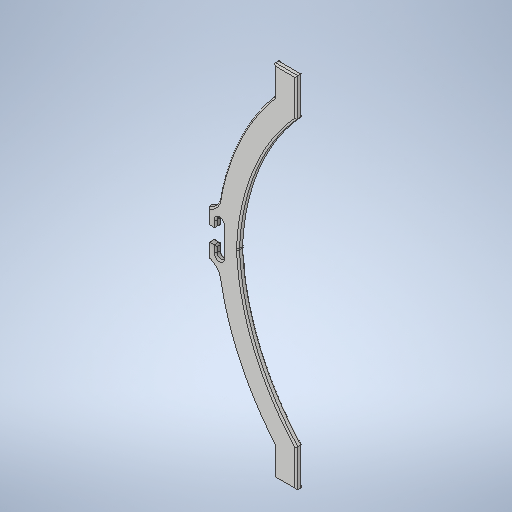
# Autodesk Inventor part: Baseplate_aussen
Saved by Autodesk Inventor 2025 (Build 290162000, 162)
## iProperties
Created: 2020-01-15
Part Number: Baseplate_aussen
Material: Generisch
Document SubType Name: Modeling
Designer: maxse
Density: 1 g/cm^3
Appearance: Vorgabe
Author: maxse
Autodesk Inventor part; units mm, degrees
(part 1 of 2)
ref_plane "YZ Plane" through (0, 0, 0) normal (1, 0, 0) x (0, 1, 0)
ref_plane "XZ Plane" through (0, 0, 0) normal (0, 1, 0) x (-1, 0, 0)
ref_plane "XY Plane" through (0, 0, 0) normal (0, 0, 1) x (1, 0, 0)
sketch "Skizze1" plane through (0, 0, 0) normal (0, 1, 0) x (-1, 0, 0)
  arc A0 (39, 0) -> (0, 95) centre (-110.879, -6.024) ccw
  line L0 (0, 95) -> (0, 120)
  line L1 (0, 120) -> (15, 120)
  line L2 (15, 120) -> (15, 100.6336)
  arc A1 (54, 0) -> (15, 100.6336) centre (-110.879, -6.024) ccw
  line L3 (39, 0) -> (54, 0)
  line L4 (0, 0) -> (39, 0)
  line L5 (59, 0) -> (59, 15)
  line L6 (59, 15) -> (52.765, 15)
  line L7 (59, 0) -> (54, 0)
  dimension "d0" = 25
  dimension "d2" = 15
  dimension "d4" = 54
  dimension "d5" = 0
  dimension "d6" = 120
  dimension "d7" = 150
  dimension "d9" = 5
  dimension "d10" = 15
  dimension "d11" = 15
  constraints: 16 end point, 6 point on circle, 3 perpendicular, 2 centre point, 2 horizontal, 2 vertical, 1 collinear, 1 concentric
  measures "d0" distance of L0.start L0.end
  measures "d2" distance of L0.end L1.end
  measures "d4" distance of L3.end L4.start
  measures "d5" distance from line of L4.start L0
  measures "d6" distance from line of L4.start L1
  measures "d7" radius of A0
  measures "d9" distance of L3.end L5.start
  measures "d10" distance of L3.end L3.start
  measures "d11" distance of L5.start L5.end
extrude "Extrusion1" add sketch "Skizze1" along normal blind 4
mirror "Spiegeln1" about plane through (-54, 0, 0) normal (0, 0, -1) of "Extrusion1"
sketch "Skizze2" plane through (0, 0, 0) normal (0, -1, 0) x (1, 0, 0)
  line L0 (-59, 15) -> (-59, -15) projected
  line L1 (-59, -5) -> (-54, -5)
  line L2 (-54, -5) -> (-54, -9.5)
  line L3 (-59, 5) -> (-54, 5)
  line L4 (-54, 5) -> (-54, 9.5)
  line L5 (-49, -9.5) -> (-49, 9.5)
  arc A0 (-49, 9.5) -> (-54, 9.5) centre (-51.5, 9.5) ccw
  arc A1 (-54, -9.5) -> (-49, -9.5) centre (-51.5, -9.5) ccw
  point P0 (0, 0)
  dimension "d15" = 10
  dimension "d16" = 5
  dimension "d17" = 10
  dimension "d18" = 5
  dimension "d19" = 5
  dimension "d20" = 24
  dimension "d21" = 4.5
  constraints: 10 end point, 4 point on circle, 4 tangent, 2 centre point, 2 horizontal, 2 point on line, 2 vertical, 1 perpendicular
  measures "d15" distance between parallel lines of L5 L0
  measures "d16" distance between parallel lines of L5 L2
  measures "d17" distance between parallel lines of L3 L1
  measures "d18" distance of L3.start L3.end
  measures "d19" distance from line of point (0, 0) L3
  measures "d21" distance from line of L1 A1.centre
extrude "Extrusion2" cut sketch "Skizze2" against normal blind 4
fillet "Rundung1" radius 10 3 edges at (-52.765, 2, -15) (-52.765, 2, 15) (-39, 2, 0)
fillet "Rundung2" radius 1 46 edges at (-7.5, 4, -120) (0, 4, -107.5) (-15, 4, -110.3168) (-7.5, 0, -120) (0, 0, -107.5) (-15, 0, -110.3168) (-54.0935, 4, -17.8718) (-38.4134, 4, -64.2123) (-54.0935, 0, -17.8718) (-38.4134, 0, -64.2123) (-38.9913, 4, 0) (-27.8012, 4, 51.1406) (-27.8012, 4, -51.1406) (-38.9913, 0, 0) (-27.8012, 0, 51.1406) (-27.8012, 0, -51.1406) (-54.0935, 4, 17.8718) (-38.4134, 4, 64.2123) (-54.0935, 0, 17.8718) (-38.4134, 0, 64.2123) (-59, 4, 10) (-59, 0, 10) (-59, 0, -10) (-59, 4, -10) (-59, 2, -5) (-59, 2, 5) (-54, 2, 5) (-54, 2, -5) (-56.5, 4, -5) (-56.5, 4, 5) (-51.5, 4, 12) (-54, 4, 7.25) (-51.5, 4, -12) (-54, 4, -7.25) (-49, 4, 0) (-51.5, 0, -12) (-54, 0, -7.25) (-51.5, 0, 12) (-54, 0, 7.25) (-49, 0, 0) (-15, 4, 110.3168) (-15, 0, 110.3168) (-7.5, 4, 120) (-7.5, 0, 120) (0, 0, 107.5) (0, 4, 107.5)
sketch "Skizze3" plane through (0, 4, 0) normal (0, 1, 0) x (1, 0, 0)
  line L0 (0, 120) -> (0, 95) projected
  arc A0 (0, 95) -> (0, -95.3865) centre (95.1198, -0.1933) ccw
  line L1 (-30.1986, 63.5083) -> (-29.9063, 64.0688)
  line L2 (-29.9063, 64.0688) -> (-28.0095, 63.0792)
  spline S0 degree 2 poles (-28.0095, 63.0792) (-27.7796, 62.9593) (-27.3619, 62.7962) (-27.2096, 62.799) knots 0 0 0 1 2 2 2
  spline S1 degree 2 poles (-27.2096, 62.799) (-27.0483, 62.8017) (-26.7987, 62.9822) (-26.69, 63.1906) knots 0 0 0 1 2 2 2
  spline S2 degree 2 poles (-26.69, 63.1906) (-26.5813, 63.399) (-26.5735, 63.957) (-26.6426, 64.2627) knots 0 0 0 1 2 2 2
  line L3 (-26.6426, 64.2627) -> (-29.1285, 65.5596)
  line L4 (-29.1285, 65.5596) -> (-28.8361, 66.12)
  line L5 (-28.8361, 66.12) -> (-24.2056, 63.7042)
  line L6 (-24.2056, 63.7042) -> (-24.4979, 63.1438)
  line L7 (-24.4979, 63.1438) -> (-26.172, 64.0172)
  spline S3 degree 2 poles (-26.172, 64.0172) (-26.0768, 63.6476) (-26.0928, 63.039) (-26.2352, 62.7659) knots 0 0 0 1 2 2 2
  spline S4 degree 2 poles (-26.2352, 62.7659) (-26.4901, 62.2774) (-27.4253, 62.0615) (-28.0396, 62.382) knots 0 0 0 1 2 2 2
  line L8 (-28.0396, 62.382) -> (-30.1986, 63.5083)
  spline S5 degree 2 poles (-30.2636, 59.1219) (-31.1157, 59.5377) (-31.6445, 60.8101) (-31.3105, 61.4947) knots 0 0 0 1 2 2 2
  spline S6 degree 2 poles (-31.3105, 61.4947) (-30.9676, 62.1975) (-29.6172, 62.535) (-28.7942, 62.1334) knots 0 0 0 1 2 2 2
  spline S7 degree 2 poles (-28.7942, 62.1334) (-27.9494, 61.7212) (-27.4186, 60.4343) (-27.7491, 59.757) knots 0 0 0 1 2 2 2
  spline S8 degree 2 poles (-27.7491, 59.757) (-28.0831, 59.0724) (-29.4152, 58.7079) (-30.2636, 59.1219) knots 0 0 0 1 2 2 2
  spline S9 degree 2 poles (-29.9776, 59.7082) (-29.3221, 59.3884) (-28.4521, 59.5545) (-28.2371, 59.9951) knots 0 0 0 1 2 2 2
  spline S10 degree 2 poles (-28.2371, 59.9951) (-28.0221, 60.4357) (-28.4248, 61.2273) (-29.0803, 61.5471) knots 0 0 0 1 2 2 2
  spline S11 degree 2 poles (-29.0803, 61.5471) (-29.7175, 61.8581) (-30.6075, 61.6972) (-30.8225, 61.2566) knots 0 0 0 1 2 2 2
  spline S12 degree 2 poles (-30.8225, 61.2566) (-31.0357, 60.8196) (-30.6257, 60.0245) (-29.9776, 59.7082) knots 0 0 0 1 2 2 2
  line L9 (-32.4885, 58.7697) -> (-32.222, 59.3429)
  line L10 (-32.222, 59.3429) -> (-27.4858, 57.1415)
  line L11 (-27.4858, 57.1415) -> (-27.7522, 56.5683)
  line L12 (-27.7522, 56.5683) -> (-32.4885, 58.7697)
  line L13 (-34.047, 55.2901) -> (-33.7916, 55.8683)
  line L14 (-33.7916, 55.8683) -> (-33.4432, 55.7144)
  spline S13 degree 2 poles (-33.4432, 55.7144) (-33.4954, 55.897) (-33.5569, 56.1589) (-33.561, 56.3202) knots 0 0 0 1 2 2 2
  spline S14 degree 2 poles (-33.561, 56.3202) (-33.5663, 56.4687) (-33.513, 56.7596) (-33.4361, 56.9338) knots 0 0 0 1 2 2 2
  spline S15 degree 2 poles (-33.4361, 56.9338) (-33.3116, 57.2155) (-32.8686, 57.5868) (-32.5688, 57.6537) knots 0 0 0 1 2 2 2
  spline S16 degree 2 poles (-32.5688, 57.6537) (-32.269, 57.7206) (-31.52, 57.6112) (-31.0864, 57.4196) knots 0 0 0 1 2 2 2
  spline S17 degree 2 poles (-31.0864, 57.4196) (-30.6342, 57.2199) (-30.0776, 56.695) (-29.9194, 56.3814) knots 0 0 0 1 2 2 2
  spline S18 degree 2 poles (-29.9194, 56.3814) (-29.7805, 56.0942) (-29.7589, 55.4512) (-29.8882, 55.1584) knots 0 0 0 1 2 2 2
  spline S19 degree 2 poles (-29.8882, 55.1584) (-30.0012, 54.9026) (-30.2847, 54.5716) (-30.4967, 54.4128) knots 0 0 0 1 2 2 2
  line L15 (-30.4967, 54.4128) -> (-29.0141, 53.7579)
  line L16 (-29.0141, 53.7579) -> (-29.2696, 53.1797)
  line L17 (-29.2696, 53.1797) -> (-34.047, 55.2901)
  line L18 (-32.9577, 55.4999) -> (-30.9748, 54.624)
  spline S20 degree 2 poles (-30.9748, 54.624) (-30.776, 54.7931) (-30.5476, 55.0997) (-30.4608, 55.2961) knots 0 0 0 1 2 2 2
  spline S21 degree 2 poles (-30.4608, 55.2961) (-30.2643, 55.7409) (-30.7088, 56.5397) (-31.3389, 56.818) knots 0 0 0 1 2 2 2
  spline S22 degree 2 poles (-31.3389, 56.818) (-31.9467, 57.0865) (-32.7582, 56.9843) (-32.9465, 56.5581) knots 0 0 0 1 2 2 2
  spline S23 degree 2 poles (-32.9465, 56.5581) (-33.0463, 56.332) (-33.0418, 55.7807) (-32.9577, 55.4999) knots 0 0 0 1 2 2 2
  spline S24 degree 2 poles (-35.1022, 52.9728) (-34.7605, 53.8049) (-33.4517, 54.3363) (-32.5896, 53.9824) knots 0 0 0 1 2 2 2
  spline S25 degree 2 poles (-32.5896, 53.9824) (-31.7425, 53.6346) (-31.1027, 52.3338) (-31.3967, 51.6179) knots 0 0 0 1 2 2 2
  spline S26 degree 2 poles (-31.3967, 51.6179) (-31.529, 51.2955) (-31.9211, 50.874) (-32.1952, 50.7719) knots 0 0 0 1 2 2 2
  spline S27 degree 2 poles (-32.1952, 50.7719) (-32.4708, 50.666) (-33.1258, 50.7028) (-33.5419, 50.8736) knots 0 0 0 1 2 2 2
  line L19 (-33.5419, 50.8736) -> (-33.8605, 51.0044)
  line L20 (-33.8605, 51.0044) -> (-32.874, 53.4071)
  spline S28 degree 2 poles (-32.874, 53.4071) (-33.4775, 53.6548) (-34.3677, 53.3108) (-34.5894, 52.771) knots 0 0 0 1 2 2 2
  spline S29 degree 2 poles (-34.5894, 52.771) (-34.6678, 52.5799) (-34.734, 52.1734) (-34.7281, 51.9958) knots 0 0 0 1 2 2 2
  spline S30 degree 2 poles (-34.7281, 51.9958) (-34.7177, 51.8076) (-34.6758, 51.5363) (-34.6451, 51.4405) knots 0 0 0 1 2 2 2
  line L21 (-34.6451, 51.4405) -> (-34.6589, 51.4067)
  line L22 (-34.6589, 51.4067) -> (-35.2961, 51.6684)
  spline S31 degree 2 poles (-35.2961, 51.6684) (-35.2958, 51.7865) (-35.2896, 52.1431) (-35.274, 52.2769) knots 0 0 0 1 2 2 2
  spline S32 degree 2 poles (-35.274, 52.2769) (-35.2535, 52.4656) (-35.1884, 52.7629) (-35.1022, 52.9728) knots 0 0 0 1 2 2 2
  spline S33 degree 2 poles (-33.1805, 51.391) (-32.9413, 51.3016) (-32.5565, 51.2575) (-32.4018, 51.3035) knots 0 0 0 1 2 2 2
  spline S34 degree 2 poles (-32.4018, 51.3035) (-32.229, 51.3508) (-31.9596, 51.6125) (-31.8626, 51.8486) knots 0 0 0 1 2 2 2
  spline S35 degree 2 poles (-31.8626, 51.8486) (-31.7672, 52.081) (-31.772, 52.464) (-31.8515, 52.6544) knots 0 0 0 1 2 2 2
  spline S36 degree 2 poles (-31.8515, 52.6544) (-31.9363, 52.8425) (-32.2145, 53.1144) (-32.428, 53.2239) knots 0 0 0 1 2 2 2
  line L23 (-32.428, 53.2239) -> (-33.1805, 51.391)
  line L24 (-33.6101, 48.1318) -> (-33.5984, 48.162)
  spline S37 degree 2 poles (-33.5984, 48.162) (-33.5533, 48.2228) (-33.4889, 48.3673) (-33.4495, 48.4694) knots 0 0 0 1 2 2 2
  spline S38 degree 2 poles (-33.4495, 48.4694) (-33.3577, 48.7076) (-33.385, 49.2565) (-33.5075, 49.547) knots 0 0 0 1 2 2 2
  line L25 (-33.5075, 49.547) -> (-35.9915, 50.5044)
  line L26 (-35.9915, 50.5044) -> (-35.7641, 51.0942)
  line L27 (-35.7641, 51.0942) -> (-32.2632, 49.7447)
  line L28 (-32.2632, 49.7447) -> (-32.4905, 49.1549)
  line L29 (-32.4905, 49.1549) -> (-33.0122, 49.3561)
  spline S39 degree 2 poles (-33.0122, 49.3561) (-32.8488, 48.9239) (-32.7995, 48.3534) (-32.8869, 48.1266) knots 0 0 0 1 2 2 2
  spline S40 degree 2 poles (-32.8869, 48.1266) (-32.9219, 48.0359) (-32.9644, 47.948) (-32.9976, 47.8957) knots 0 0 0 1 2 2 2
  line L30 (-32.9976, 47.8957) -> (-33.6101, 48.1318)
  line L31 (-33.6727, 43.3761) -> (-33.662, 43.4067)
  spline S41 degree 2 poles (-33.662, 43.4067) (-33.6034, 43.4764) (-33.4458, 43.7561) (-33.4044, 43.8747) knots 0 0 0 1 2 2 2
  spline S42 degree 2 poles (-33.4044, 43.8747) (-33.2737, 44.2497) (-33.4983, 44.6884) (-33.9421, 44.8432) knots 0 0 0 1 2 2 2
  line L32 (-33.9421, 44.8432) -> (-34.0607, 44.8845)
  line L33 (-34.0607, 44.8845) -> (-34.4049, 43.8975)
  line L34 (-34.4049, 43.8975) -> (-34.8985, 44.0695)
  line L35 (-34.8985, 44.0695) -> (-34.5609, 45.0375)
  line L36 (-34.5609, 45.0375) -> (-37.6102, 46.1008)
  line L37 (-37.6102, 46.1008) -> (-37.4021, 46.6976)
  line L38 (-37.4021, 46.6976) -> (-34.3528, 45.6344)
  line L39 (-34.3528, 45.6344) -> (-34.2127, 46.0361)
  line L40 (-34.2127, 46.0361) -> (-33.7192, 45.864)
  line L41 (-33.7192, 45.864) -> (-33.8593, 45.4623)
  line L42 (-33.8593, 45.4623) -> (-33.7407, 45.4209)
  spline S43 degree 2 poles (-33.7407, 45.4209) (-33.1056, 45.1995) (-32.6546, 44.3514) (-32.8547, 43.7775) knots 0 0 0 1 2 2 2
  spline S44 degree 2 poles (-32.8547, 43.7775) (-32.9121, 43.6129) (-33.0573, 43.3074) (-33.1256, 43.1853) knots 0 0 0 1 2 2 2
  line L43 (-33.1256, 43.1853) -> (-33.6727, 43.3761)
  spline S45 degree 2 poles (-37.3148, 41.0423) (-38.2166, 41.335) (-38.9178, 42.5212) (-38.6826, 43.2457) knots 0 0 0 1 2 2 2
  spline S46 degree 2 poles (-38.6826, 43.2457) (-38.4411, 43.9895) (-37.151, 44.5122) (-36.28, 44.2294) knots 0 0 0 1 2 2 2
  spline S47 degree 2 poles (-36.28, 44.2294) (-35.386, 43.9391) (-34.6808, 42.7389) (-34.9135, 42.0221) knots 0 0 0 1 2 2 2
  spline S48 degree 2 poles (-34.9135, 42.0221) (-35.1488, 41.2975) (-36.4169, 40.7507) (-37.3148, 41.0423) knots 0 0 0 1 2 2 2
  spline S49 degree 2 poles (-37.1134, 41.6627) (-36.4197, 41.4375) (-35.5813, 41.7234) (-35.4299, 42.1897) knots 0 0 0 1 2 2 2
  spline S50 degree 2 poles (-35.4299, 42.1897) (-35.2785, 42.656) (-35.7878, 43.3837) (-36.4815, 43.6089) knots 0 0 0 1 2 2 2
  spline S51 degree 2 poles (-36.4815, 43.6089) (-37.1559, 43.8279) (-38.0148, 43.5444) (-38.1662, 43.0781) knots 0 0 0 1 2 2 2
  spline S52 degree 2 poles (-38.1662, 43.0781) (-38.3163, 42.6156) (-37.7993, 41.8854) (-37.1134, 41.6627) knots 0 0 0 1 2 2 2
  line L44 (-36.9101, 38.2097) -> (-36.9008, 38.2408)
  spline S53 degree 2 poles (-36.9008, 38.2408) (-36.8604, 38.3048) (-36.8072, 38.4538) (-36.7757, 38.5586) knots 0 0 0 1 2 2 2
  spline S54 degree 2 poles (-36.7757, 38.5586) (-36.7023, 38.8031) (-36.7711, 39.3484) (-36.9154, 39.6286) knots 0 0 0 1 2 2 2
  line L45 (-36.9154, 39.6286) -> (-39.4649, 40.3945)
  line L46 (-39.4649, 40.3945) -> (-39.2831, 40.9999)
  line L47 (-39.2831, 40.9999) -> (-35.6897, 39.9204)
  line L48 (-35.6897, 39.9204) -> (-35.8715, 39.315)
  line L49 (-35.8715, 39.315) -> (-36.4071, 39.4759)
  spline S55 degree 2 poles (-36.4071, 39.4759) (-36.2112, 39.0575) (-36.1187, 38.4923) (-36.1886, 38.2595) knots 0 0 0 1 2 2 2
  spline S56 degree 2 poles (-36.1886, 38.2595) (-36.2166, 38.1664) (-36.2524, 38.0756) (-36.2815, 38.0209) knots 0 0 0 1 2 2 2
  line L50 (-36.2815, 38.0209) -> (-36.9101, 38.2097)
  spline S57 degree 2 poles (-41.0374, 35.2117) (-40.9436, 35.5725) (-40.574, 36.1085) (-40.3199, 36.2644) knots 0 0 0 1 2 2 2
  spline S58 degree 2 poles (-40.3199, 36.2644) (-40.0708, 36.4173) (-39.4825, 36.4904) (-39.1805, 36.4118) knots 0 0 0 1 2 2 2
  spline S59 degree 2 poles (-39.1805, 36.4118) (-38.7884, 36.3099) (-38.2387, 35.719) (-38.1466, 35.268) knots 0 0 0 1 2 2 2
  line L51 (-38.1466, 35.268) -> (-38.127, 35.2629)
  spline S60 degree 2 poles (-38.127, 35.2629) (-37.8264, 35.5657) (-37.2425, 35.7823) (-36.8739, 35.6865) knots 0 0 0 1 2 2 2
  spline S61 degree 2 poles (-36.8739, 35.6865) (-36.3288, 35.5447) (-35.8136, 34.5316) (-35.9788, 33.8963) knots 0 0 0 1 2 2 2
  spline S62 degree 2 poles (-35.9788, 33.8963) (-36.1501, 33.2375) (-37.0472, 32.6209) (-37.5884, 32.7616) knots 0 0 0 1 2 2 2
  spline S63 degree 2 poles (-37.5884, 32.7616) (-37.9139, 32.8462) (-38.4502, 33.3918) (-38.5378, 33.7956) knots 0 0 0 1 2 2 2
  line L52 (-38.5378, 33.7956) -> (-38.5574, 33.8007)
  spline S64 degree 2 poles (-38.5574, 33.8007) (-38.8636, 33.4281) (-39.5415, 33.1397) (-39.9886, 33.2559) knots 0 0 0 1 2 2 2
  spline S65 degree 2 poles (-39.9886, 33.2559) (-40.6082, 33.417) (-41.2128, 34.5372) (-41.0374, 35.2117) knots 0 0 0 1 2 2 2
  spline S66 degree 2 poles (-39.878, 33.9389) (-39.5799, 33.8614) (-39.1658, 34.0049) (-38.8988, 34.2913) knots 0 0 0 1 2 2 2
  spline S67 degree 2 poles (-38.8988, 34.2913) (-38.8075, 34.3848) (-38.5665, 34.7157) (-38.4122, 34.9226) knots 0 0 0 1 2 2 2
  spline S68 degree 2 poles (-38.4122, 34.9226) (-38.5194, 35.2351) (-38.9704, 35.6581) (-39.3037, 35.7447) knots 0 0 0 1 2 2 2
  spline S69 degree 2 poles (-39.3037, 35.7447) (-39.7429, 35.8589) (-40.4531, 35.4784) (-40.5571, 35.0784) knots 0 0 0 1 2 2 2
  spline S70 degree 2 poles (-40.5571, 35.0784) (-40.6632, 34.6706) (-40.3015, 34.049) (-39.878, 33.9389) knots 0 0 0 1 2 2 2
  spline S71 degree 2 poles (-37.4311, 33.3989) (-37.1056, 33.3143) (-36.5571, 33.6364) (-36.4562, 34.0246) knots 0 0 0 1 2 2 2
  spline S72 degree 2 poles (-36.4562, 34.0246) (-36.3644, 34.3775) (-36.6353, 34.9295) (-36.9687, 35.0161) knots 0 0 0 1 2 2 2
  spline S73 degree 2 poles (-36.9687, 35.0161) (-37.2079, 35.0783) (-37.6014, 34.9336) (-37.7948, 34.7369) knots 0 0 0 1 2 2 2
  spline S74 degree 2 poles (-37.7948, 34.7369) (-37.8752, 34.6532) (-38.1755, 34.2875) (-38.2742, 34.1331) knots 0 0 0 1 2 2 2
  spline S75 degree 2 poles (-38.2742, 34.1331) (-38.132, 33.7947) (-37.7252, 33.4754) (-37.4311, 33.3989) knots 0 0 0 1 2 2 2
  spline S76 degree 2 poles (-40.6166, 29.5675) (-40.9916, 29.6544) (-41.5695, 30.0503) (-41.7342, 30.3089) knots 0 0 0 1 2 2 2
  spline S77 degree 2 poles (-41.7342, 30.3089) (-41.9089, 30.5782) (-42.0155, 31.1769) (-41.9396, 31.5045) knots 0 0 0 1 2 2 2
  spline S78 degree 2 poles (-41.9396, 31.5045) (-41.8637, 31.8321) (-41.5173, 32.3217) (-41.2487, 32.4757) knots 0 0 0 1 2 2 2
  spline S79 degree 2 poles (-41.2487, 32.4757) (-40.9257, 32.667) (-39.9717, 32.7454) (-39.3244, 32.5954) knots 0 0 0 1 2 2 2
  spline S80 degree 2 poles (-39.3244, 32.5954) (-38.6888, 32.4482) (-37.7269, 31.9508) (-37.411, 31.5906) knots 0 0 0 1 2 2 2
  spline S81 degree 2 poles (-37.411, 31.5906) (-37.1013, 31.2401) (-36.8807, 30.3073) (-37.0079, 29.7586) knots 0 0 0 1 2 2 2
  spline S82 degree 2 poles (-37.0079, 29.7586) (-37.0454, 29.5968) (-37.1428, 29.3199) (-37.203, 29.2215) knots 0 0 0 1 2 2 2
  line L53 (-37.203, 29.2215) -> (-37.8307, 29.367)
  line L54 (-37.8307, 29.367) -> (-37.8243, 29.3946)
  spline S83 degree 2 poles (-37.8243, 29.3946) (-37.7558, 29.4744) (-37.5961, 29.7868) (-37.5522, 29.9762) knots 0 0 0 1 2 2 2
  spline S84 degree 2 poles (-37.5522, 29.9762) (-37.4114, 30.5841) (-38.0595, 31.5204) (-38.8483, 31.7781) knots 0 0 0 1 2 2 2
  spline S85 degree 2 poles (-38.8483, 31.7781) (-38.7404, 31.5077) (-38.6762, 30.977) (-38.7439, 30.6849) knots 0 0 0 1 2 2 2
  spline S86 degree 2 poles (-38.7439, 30.6849) (-38.8098, 30.4007) (-39.023, 30.001) (-39.2507, 29.8083) knots 0 0 0 1 2 2 2
  spline S87 degree 2 poles (-39.2507, 29.8083) (-39.5142, 29.5865) (-40.1982, 29.4705) (-40.6166, 29.5675) knots 0 0 0 1 2 2 2
  spline S88 degree 2 poles (-40.4906, 30.237) (-40.1906, 30.1675) (-39.7474, 30.2312) (-39.5651, 30.372) knots 0 0 0 1 2 2 2
  spline S89 degree 2 poles (-39.5651, 30.372) (-39.4323, 30.4784) (-39.2902, 30.7866) (-39.2508, 30.9563) knots 0 0 0 1 2 2 2
  spline S90 degree 2 poles (-39.2508, 30.9563) (-39.1978, 31.1852) (-39.2362, 31.6475) (-39.318, 31.8869) knots 0 0 0 1 2 2 2
  spline S91 degree 2 poles (-39.318, 31.8869) (-39.3882, 31.9073) (-39.5205, 31.9463) (-39.6232, 31.9701) knots 0 0 0 1 2 2 2
  spline S92 degree 2 poles (-39.6232, 31.9701) (-40.1284, 32.0872) (-40.7939, 32.0334) (-40.9905, 31.9209) knots 0 0 0 1 2 2 2
  spline S93 degree 2 poles (-40.9905, 31.9209) (-41.1764, 31.8184) (-41.3683, 31.5468) (-41.4076, 31.3771) knots 0 0 0 1 2 2 2
  spline S94 degree 2 poles (-41.4076, 31.3771) (-41.4991, 30.9823) (-41.0511, 30.3669) (-40.4906, 30.237) knots 0 0 0 1 2 2 2
  line L55 (-43.1711, 25.0919) -> (-41.04, 24.6736)
  spline S95 degree 2 poles (-41.04, 24.6736) (-40.7856, 24.6236) (-40.3444, 24.5783) (-40.2126, 24.6185) knots 0 0 0 1 2 2 2
  spline S96 degree 2 poles (-40.2126, 24.6185) (-40.0689, 24.6564) (-39.8941, 24.8739) (-39.8527, 25.0847) knots 0 0 0 1 2 2 2
  spline S97 degree 2 poles (-39.8527, 25.0847) (-39.8152, 25.2755) (-39.964, 25.7589) (-40.1414, 26.0332) knots 0 0 0 1 2 2 2
  spline S98 degree 2 poles (-40.1414, 26.0332) (-40.1978, 26.0402) (-40.3544, 26.0627) (-40.4578, 26.083) knots 0 0 0 1 2 2 2
  line L56 (-40.4578, 26.083) -> (-42.8832, 26.559)
  line L57 (-42.8832, 26.559) -> (-42.7614, 27.1793)
  line L58 (-42.7614, 27.1793) -> (-40.6303, 26.761)
  spline S99 degree 2 poles (-40.6303, 26.761) (-40.3758, 26.711) (-39.9346, 26.6657) (-39.8029, 26.7059) knots 0 0 0 1 2 2 2
  spline S100 degree 2 poles (-39.8029, 26.7059) (-39.6592, 26.7438) (-39.4843, 26.9613) (-39.443, 27.1721) knots 0 0 0 1 2 2 2
  spline S101 degree 2 poles (-39.443, 27.1721) (-39.4039, 27.3709) (-39.5678, 27.8614) (-39.722, 28.1064) knots 0 0 0 1 2 2 2
  line L59 (-39.722, 28.1064) -> (-42.4734, 28.6464)
  line L60 (-42.4734, 28.6464) -> (-42.3517, 29.2667)
  line L61 (-42.3517, 29.2667) -> (-38.6699, 28.544)
  line L62 (-38.6699, 28.544) -> (-38.7917, 27.9237)
  line L63 (-38.7917, 27.9237) -> (-39.1972, 28.0033)
  spline S102 degree 2 poles (-39.1972, 28.0033) (-39.0023, 27.7132) (-38.8295, 27.1838) (-38.8857, 26.8975) knots 0 0 0 1 2 2 2
  spline S103 degree 2 poles (-38.8857, 26.8975) (-38.9497, 26.5715) (-39.347, 26.1251) (-39.7108, 26.0602) knots 0 0 0 1 2 2 2
  spline S104 degree 2 poles (-39.7108, 26.0602) (-39.4521, 25.7162) (-39.2346, 25.1202) (-39.2955, 24.8101) knots 0 0 0 1 2 2 2
  spline S105 degree 2 poles (-39.2955, 24.8101) (-39.3423, 24.5716) (-39.5659, 24.2108) (-39.761, 24.1004) knots 0 0 0 1 2 2 2
  spline S106 degree 2 poles (-39.761, 24.1004) (-39.9569, 23.9861) (-40.4898, 23.9214) (-40.8675, 23.9956) knots 0 0 0 1 2 2 2
  line L64 (-40.8675, 23.9956) -> (-43.2929, 24.4716)
  line L65 (-43.2929, 24.4716) -> (-43.1711, 25.0919)
  line L66 (-44.0927, 19.3927) -> (-41.9462, 19.0623)
  spline S107 degree 2 poles (-41.9462, 19.0623) (-41.6899, 19.0228) (-41.2472, 18.9957) (-41.1172, 19.0412) knots 0 0 0 1 2 2 2
  spline S108 degree 2 poles (-41.1172, 19.0412) (-40.9752, 19.085) (-40.8094, 19.3095) (-40.7767, 19.5218) knots 0 0 0 1 2 2 2
  spline S109 degree 2 poles (-40.7767, 19.5218) (-40.7471, 19.714) (-40.9156, 20.1909) (-41.1041, 20.4577) knots 0 0 0 1 2 2 2
  spline S110 degree 2 poles (-41.1041, 20.4577) (-41.1608, 20.4623) (-41.3182, 20.4783) (-41.4223, 20.4944) knots 0 0 0 1 2 2 2
  line L67 (-41.4223, 20.4944) -> (-43.8652, 20.8705)
  line L68 (-43.8652, 20.8705) -> (-43.769, 21.4952)
  line L69 (-43.769, 21.4952) -> (-41.6225, 21.1647)
  spline S111 degree 2 poles (-41.6225, 21.1647) (-41.3662, 21.1253) (-40.9235, 21.0981) (-40.7935, 21.1437) knots 0 0 0 1 2 2 2
  spline S112 degree 2 poles (-40.7935, 21.1437) (-40.6515, 21.1874) (-40.4857, 21.412) (-40.453, 21.6242) knots 0 0 0 1 2 2 2
  spline S113 degree 2 poles (-40.453, 21.6242) (-40.4222, 21.8245) (-40.6061, 22.3078) (-40.7702, 22.5463) knots 0 0 0 1 2 2 2
  line L70 (-40.7702, 22.5463) -> (-43.5415, 22.9729)
  line L71 (-43.5415, 22.9729) -> (-43.4453, 23.5977)
  line L72 (-43.4453, 23.5977) -> (-39.737, 23.0267)
  line L73 (-39.737, 23.0267) -> (-39.8331, 22.402)
  line L74 (-39.8331, 22.402) -> (-40.2416, 22.4649)
  spline S114 degree 2 poles (-40.2416, 22.4649) (-40.0349, 22.183) (-39.8406, 21.6611) (-39.885, 21.3728) knots 0 0 0 1 2 2 2
  spline S115 degree 2 poles (-39.885, 21.3728) (-39.9356, 21.0444) (-40.3142, 20.5821) (-40.675, 20.5023) knots 0 0 0 1 2 2 2
  spline S116 degree 2 poles (-40.675, 20.5023) (-40.4024, 20.1693) (-40.1606, 19.5827) (-40.2087, 19.2703) knots 0 0 0 1 2 2 2
  spline S117 degree 2 poles (-40.2087, 19.2703) (-40.2457, 19.03) (-40.4543, 18.6604) (-40.6447, 18.5421) knots 0 0 0 1 2 2 2
  spline S118 degree 2 poles (-40.6447, 18.5421) (-40.8357, 18.4199) (-41.3656, 18.3333) (-41.746, 18.3919) knots 0 0 0 1 2 2 2
  line L75 (-41.746, 18.3919) -> (-44.1889, 18.768)
  line L76 (-44.1889, 18.768) -> (-44.0927, 19.3927)
  line L77 (-43.4887, 16.5567) -> (-45.5547, 17.7633)
  line L78 (-45.5547, 17.7633) -> (-45.4937, 18.2497)
  line L79 (-45.4937, 18.2497) -> (-43.3843, 17.3889)
  line L80 (-43.3843, 17.3889) -> (-43.4887, 16.5567)
  spline S119 degree 2 poles (-43.4508, 10.6171) (-43.81, 10.649) (-44.403, 10.9337) (-44.6103, 11.1637) knots 0 0 0 1 2 2 2
  spline S120 degree 2 poles (-44.6103, 11.1637) (-44.8176, 11.3937) (-45.0243, 12.0426) (-44.9898, 12.43) knots 0 0 0 1 2 2 2
  spline S121 degree 2 poles (-44.9898, 12.43) (-44.9582, 12.7852) (-44.739, 13.4654) (-44.5912, 13.7085) knots 0 0 0 1 2 2 2
  line L81 (-44.5912, 13.7085) -> (-43.8849, 13.6456)
  line L82 (-43.8849, 13.6456) -> (-43.8893, 13.5972)
  spline S122 degree 2 poles (-43.8893, 13.5972) (-43.9526, 13.5255) (-44.1234, 13.2519) (-44.2034, 13.0841) knots 0 0 0 1 2 2 2
  spline S123 degree 2 poles (-44.2034, 13.0841) (-44.2896, 12.8925) (-44.3954, 12.5724) (-44.4137, 12.3665) knots 0 0 0 1 2 2 2
  spline S124 degree 2 poles (-44.4137, 12.3665) (-44.4317, 12.1648) (-44.3202, 11.7724) (-44.175, 11.6212) knots 0 0 0 1 2 2 2
  spline S125 degree 2 poles (-44.175, 11.6212) (-44.0368, 11.4828) (-43.6528, 11.3184) (-43.3864, 11.2947) knots 0 0 0 1 2 2 2
  spline S126 degree 2 poles (-43.3864, 11.2947) (-43.12, 11.271) (-42.7681, 11.3861) (-42.6429, 11.5133) knots 0 0 0 1 2 2 2
  spline S127 degree 2 poles (-42.6429, 11.5133) (-42.5052, 11.6434) (-42.3629, 12.0538) (-42.3402, 12.3081) knots 0 0 0 1 2 2 2
  spline S128 degree 2 poles (-42.3402, 12.3081) (-42.3158, 12.5825) (-42.3521, 13.1349) (-42.3737, 13.3036) knots 0 0 0 1 2 2 2
  line L83 (-42.3737, 13.3036) -> (-39.8068, 13.0751)
  line L84 (-39.8068, 13.0751) -> (-40.0501, 10.3428)
  line L85 (-40.0501, 10.3428) -> (-40.6353, 10.3949)
  line L86 (-40.6353, 10.3949) -> (-40.4492, 12.4855)
  line L87 (-40.4492, 12.4855) -> (-41.777, 12.6037)
  spline S129 degree 2 poles (-41.777, 12.6037) (-41.7716, 12.4812) (-41.7803, 12.246) (-41.789, 12.1492) knots 0 0 0 1 2 2 2
  spline S130 degree 2 poles (-41.789, 12.1492) (-41.8231, 11.7657) (-41.9953, 11.2482) (-42.2025, 11.0226) knots 0 0 0 1 2 2 2
  spline S131 degree 2 poles (-42.2025, 11.0226) (-42.41, 10.7929) (-42.9988, 10.5768) (-43.4508, 10.6171) knots 0 0 0 1 2 2 2
  spline S132 degree 2 poles (-45.2942, 8.5374) (-45.271, 8.9094) (-45.0106, 9.5063) (-44.7911, 9.7078) knots 0 0 0 1 2 2 2
  spline S133 degree 2 poles (-44.7911, 9.7078) (-44.5758, 9.9055) (-44.0122, 10.0897) (-43.7008, 10.0703) knots 0 0 0 1 2 2 2
  spline S134 degree 2 poles (-43.7008, 10.0703) (-43.2964, 10.0452) (-42.6439, 9.5702) (-42.4674, 9.1451) knots 0 0 0 1 2 2 2
  line L88 (-42.4674, 9.1451) -> (-42.4471, 9.1439)
  spline S135 degree 2 poles (-42.4471, 9.1439) (-42.2099, 9.4986) (-41.6782, 9.8228) (-41.2981, 9.7991) knots 0 0 0 1 2 2 2
  spline S136 degree 2 poles (-41.2981, 9.7991) (-40.736, 9.7642) (-40.0366, 8.8681) (-40.0773, 8.213) knots 0 0 0 1 2 2 2
  spline S137 degree 2 poles (-40.0773, 8.213) (-40.1196, 7.5336) (-40.8824, 6.7569) (-41.4404, 6.7916) knots 0 0 0 1 2 2 2
  spline S138 degree 2 poles (-41.4404, 6.7916) (-41.7761, 6.8125) (-42.4068, 7.2455) (-42.57, 7.6251) knots 0 0 0 1 2 2 2
  line L89 (-42.57, 7.6251) -> (-42.5902, 7.6263)
  spline S139 degree 2 poles (-42.5902, 7.6263) (-42.8196, 7.2022) (-43.4298, 6.7895) (-43.8908, 6.8181) knots 0 0 0 1 2 2 2
  spline S140 degree 2 poles (-43.8908, 6.8181) (-44.5298, 6.8579) (-45.3374, 7.8418) (-45.2942, 8.5374) knots 0 0 0 1 2 2 2
  spline S141 degree 2 poles (-43.9128, 7.5096) (-43.6055, 7.4905) (-43.2264, 7.7105) (-43.019, 8.0427) knots 0 0 0 1 2 2 2
  spline S142 degree 2 poles (-43.019, 8.0427) (-42.9473, 8.1519) (-42.774, 8.5228) (-42.6621, 8.7553) knots 0 0 0 1 2 2 2
  spline S143 degree 2 poles (-42.6621, 8.7553) (-42.827, 9.0417) (-43.3505, 9.3706) (-43.6943, 9.3919) knots 0 0 0 1 2 2 2
  spline S144 degree 2 poles (-43.6943, 9.3919) (-44.1472, 9.4201) (-44.7716, 8.9109) (-44.7972, 8.4984) knots 0 0 0 1 2 2 2
  spline S145 degree 2 poles (-44.7972, 8.4984) (-44.8234, 8.0778) (-44.3496, 7.5368) (-43.9128, 7.5096) knots 0 0 0 1 2 2 2
  spline S146 degree 2 poles (-41.4078, 7.4473) (-41.0721, 7.4264) (-40.5953, 7.8474) (-40.5704, 8.2477) knots 0 0 0 1 2 2 2
  spline S147 degree 2 poles (-40.5704, 8.2477) (-40.5478, 8.6117) (-40.9193, 9.1017) (-41.263, 9.123) knots 0 0 0 1 2 2 2
  spline S148 degree 2 poles (-41.263, 9.123) (-41.5097, 9.1384) (-41.8683, 8.9211) (-42.0206, 8.6911) knots 0 0 0 1 2 2 2
  spline S149 degree 2 poles (-42.0206, 8.6911) (-42.0835, 8.5935) (-42.3083, 8.1772) (-42.3758, 8.0068) knots 0 0 0 1 2 2 2
  spline S150 degree 2 poles (-42.3758, 8.0068) (-42.1714, 7.7018) (-41.7111, 7.4661) (-41.4078, 7.4473) knots 0 0 0 1 2 2 2
  line L90 (-45.4474, 1.9483) -> (-43.2765, 1.8871)
  spline S151 degree 2 poles (-43.2765, 1.8871) (-43.0173, 1.8797) (-42.5746, 1.9078) (-42.4513, 1.9692) knots 0 0 0 1 2 2 2
  spline S152 degree 2 poles (-42.4513, 1.9692) (-42.3158, 2.0302) (-42.1792, 2.2736) (-42.1732, 2.4883) knots 0 0 0 1 2 2 2
  spline S153 degree 2 poles (-42.1732, 2.4883) (-42.1677, 2.6827) (-42.3941, 3.1349) (-42.6143, 3.3763) knots 0 0 0 1 2 2 2
  spline S154 degree 2 poles (-42.6143, 3.3763) (-42.6711, 3.3738) (-42.8293, 3.3702) (-42.9346, 3.3731) knots 0 0 0 1 2 2 2
  line L91 (-42.9346, 3.3731) -> (-45.4052, 3.4429)
  line L92 (-45.4052, 3.4429) -> (-45.3874, 4.0747)
  line L93 (-45.3874, 4.0747) -> (-43.2164, 4.0134)
  spline S155 degree 2 poles (-43.2164, 4.0134) (-42.9572, 4.0061) (-42.5146, 4.0342) (-42.3913, 4.0955) knots 0 0 0 1 2 2 2
  spline S156 degree 2 poles (-42.3913, 4.0955) (-42.2558, 4.1566) (-42.1192, 4.4) (-42.1131, 4.6146) knots 0 0 0 1 2 2 2
  spline S157 degree 2 poles (-42.1131, 4.6146) (-42.1074, 4.8172) (-42.3499, 5.2739) (-42.5424, 5.4902) knots 0 0 0 1 2 2 2
  line L94 (-42.5424, 5.4902) -> (-45.3452, 5.5693)
  line L95 (-45.3452, 5.5693) -> (-45.3274, 6.2011)
  line L96 (-45.3274, 6.2011) -> (-41.5768, 6.0952)
  line L97 (-41.5768, 6.0952) -> (-41.5947, 5.4634)
  line L98 (-41.5947, 5.4634) -> (-42.0078, 5.4751)
  spline S158 degree 2 poles (-42.0078, 5.4751) (-41.7677, 5.221) (-41.5101, 4.7273) (-41.5183, 4.4357) knots 0 0 0 1 2 2 2
  spline S159 degree 2 poles (-41.5183, 4.4357) (-41.5277, 4.1036) (-41.8459, 3.5978) (-42.194, 3.4738) knots 0 0 0 1 2 2 2
  spline S160 degree 2 poles (-42.194, 3.4738) (-41.8821, 3.1772) (-41.5694, 2.6253) (-41.5783, 2.3093) knots 0 0 0 1 2 2 2
  spline S161 degree 2 poles (-41.5783, 2.3093) (-41.5852, 2.0663) (-41.7462, 1.6736) (-41.9205, 1.5326) knots 0 0 0 1 2 2 2
  spline S162 degree 2 poles (-41.9205, 1.5326) (-42.0948, 1.3876) (-42.6098, 1.2359) (-42.9946, 1.2468) knots 0 0 0 1 2 2 2
  line L99 (-42.9946, 1.2468) -> (-45.4652, 1.3165)
  line L100 (-45.4652, 1.3165) -> (-45.4474, 1.9483)
  line L101 (-45.4168, -3.8248) -> (-43.2452, -3.7968)
  spline S163 degree 2 poles (-43.2452, -3.7968) (-42.9859, -3.7935) (-42.5448, -3.7473) (-42.4241, -3.6809) knots 0 0 0 1 2 2 2
  spline S164 degree 2 poles (-42.4241, -3.6809) (-42.2912, -3.6144) (-42.1647, -3.3656) (-42.1675, -3.1509) knots 0 0 0 1 2 2 2
  spline S165 degree 2 poles (-42.1675, -3.1509) (-42.17, -2.9564) (-42.4148, -2.5138) (-42.6447, -2.2817) knots 0 0 0 1 2 2 2
  spline S166 degree 2 poles (-42.6447, -2.2817) (-42.7013, -2.2865) (-42.8592, -2.2966) (-42.9646, -2.298) knots 0 0 0 1 2 2 2
  line L102 (-42.9646, -2.298) -> (-45.436, -2.3297)
  line L103 (-45.436, -2.3297) -> (-45.4441, -1.6977)
  line L104 (-45.4441, -1.6977) -> (-43.2725, -1.6698)
  spline S167 degree 2 poles (-43.2725, -1.6698) (-43.0132, -1.6665) (-42.5721, -1.6203) (-42.4514, -1.5539) knots 0 0 0 1 2 2 2
  spline S168 degree 2 poles (-42.4514, -1.5539) (-42.3185, -1.4873) (-42.1921, -1.2385) (-42.1948, -1.0238) knots 0 0 0 1 2 2 2
  spline S169 degree 2 poles (-42.1948, -1.0238) (-42.1974, -0.8212) (-42.4585, -0.3748) (-42.6597, -0.1667) knots 0 0 0 1 2 2 2
  line L105 (-42.6597, -0.1667) -> (-45.4634, -0.2027)
  line L106 (-45.4634, -0.2027) -> (-45.4715, 0.4294)
  line L107 (-45.4715, 0.4294) -> (-41.7198, 0.4776)
  line L108 (-41.7198, 0.4776) -> (-41.7116, -0.1545)
  line L109 (-41.7116, -0.1545) -> (-42.1249, -0.1598)
  spline S170 degree 2 poles (-42.1249, -0.1598) (-41.8746, -0.4038) (-41.5969, -0.8864) (-41.5931, -1.1782) knots 0 0 0 1 2 2 2
  spline S171 degree 2 poles (-41.5931, -1.1782) (-41.5889, -1.5104) (-41.8861, -2.0288) (-42.2288, -2.167) knots 0 0 0 1 2 2 2
  spline S172 degree 2 poles (-42.2288, -2.167) (-41.905, -2.4505) (-41.5698, -2.9892) (-41.5658, -3.3052) knots 0 0 0 1 2 2 2
  spline S173 degree 2 poles (-41.5658, -3.3052) (-41.5627, -3.5483) (-41.7075, -3.9473) (-41.8758, -4.0953) knots 0 0 0 1 2 2 2
  spline S174 degree 2 poles (-41.8758, -4.0953) (-42.044, -4.2474) (-42.5524, -4.4201) (-42.9372, -4.425) knots 0 0 0 1 2 2 2
  line L110 (-42.9372, -4.425) -> (-45.4087, -4.4568)
  line L111 (-45.4087, -4.4568) -> (-45.4168, -3.8248)
  spline S175 degree 2 poles (-44.7441, -9.5508) (-44.8054, -9.4775) (-45.0236, -9.2311) (-45.0917, -9.1135) knots 0 0 0 1 2 2 2
  spline S176 degree 2 poles (-45.0917, -9.1135) (-45.1909, -8.9532) (-45.3031, -8.6475) (-45.3205, -8.3644) knots 0 0 0 1 2 2 2
  spline S177 degree 2 poles (-45.3205, -8.3644) (-45.3347, -8.1339) (-45.1865, -7.7066) (-45.0384, -7.5392) knots 0 0 0 1 2 2 2
  spline S178 degree 2 poles (-45.0384, -7.5392) (-44.894, -7.3801) (-44.4522, -7.1702) (-44.2015, -7.1548) knots 0 0 0 1 2 2 2
  spline S179 degree 2 poles (-44.2015, -7.1548) (-43.8133, -7.1309) (-43.2431, -7.4246) (-43.0634, -7.7708) knots 0 0 0 1 2 2 2
  spline S180 degree 2 poles (-43.0634, -7.7708) (-42.8984, -8.0772) (-42.7364, -8.9279) (-42.6775, -9.4236) knots 0 0 0 1 2 2 2
  line L112 (-42.6775, -9.4236) -> (-42.5562, -9.4161)
  spline S181 degree 2 poles (-42.5562, -9.4161) (-42.3378, -9.4027) (-42.075, -9.2525) (-42.0057, -9.1265) knots 0 0 0 1 2 2 2
  spline S182 degree 2 poles (-42.0057, -9.1265) (-41.9363, -9.0004) (-41.9092, -8.6496) (-41.9206, -8.4636) knots 0 0 0 1 2 2 2
  spline S183 degree 2 poles (-41.9206, -8.4636) (-41.9341, -8.2452) (-42.0999, -7.6627) (-42.2434, -7.3752) knots 0 0 0 1 2 2 2
  line L113 (-42.2434, -7.3752) -> (-42.2456, -7.3388)
  line L114 (-42.2456, -7.3388) -> (-41.6026, -7.2992)
  spline S184 degree 2 poles (-41.6026, -7.2992) (-41.5434, -7.4701) (-41.382, -8.1138) (-41.3623, -8.4333) knots 0 0 0 1 2 2 2
  spline S185 degree 2 poles (-41.3623, -8.4333) (-41.3384, -8.8215) (-41.4271, -9.3588) (-41.5718, -9.5788) knots 0 0 0 1 2 2 2
  spline S186 degree 2 poles (-41.5718, -9.5788) (-41.7128, -9.7945) (-42.1897, -10.0268) (-42.5416, -10.0485) knots 0 0 0 1 2 2 2
  line L115 (-42.5416, -10.0485) -> (-45.1016, -10.2061)
  line L116 (-45.1016, -10.2061) -> (-45.1404, -9.5753)
  line L117 (-45.1404, -9.5753) -> (-44.7441, -9.5508)
  line L118 (-44.2183, -9.5185) -> (-43.179, -9.4545)
  spline S187 degree 2 poles (-43.179, -9.4545) (-43.2131, -9.2292) (-43.324, -8.55) (-43.4019, -8.3396) knots 0 0 0 1 2 2 2
  spline S188 degree 2 poles (-43.4019, -8.3396) (-43.4942, -8.0936) (-43.8338, -7.7857) (-44.1169, -7.8032) knots 0 0 0 1 2 2 2
  spline S189 degree 2 poles (-44.1169, -7.8032) (-44.4404, -7.8231) (-44.7456, -8.2072) (-44.7242, -8.555) knots 0 0 0 1 2 2 2
  spline S190 degree 2 poles (-44.7242, -8.555) (-44.706, -8.8503) (-44.4214, -9.3199) (-44.2183, -9.5185) knots 0 0 0 1 2 2 2
  line L119 (-44.7776, -14.0253) -> (-44.8331, -13.3957)
  line L120 (-44.8331, -13.3957) -> (-42.702, -13.2077)
  spline S191 degree 2 poles (-42.702, -13.2077) (-42.4437, -13.1849) (-42.004, -13.0974) (-41.8772, -13.013) knots 0 0 0 1 2 2 2
  spline S192 degree 2 poles (-41.8772, -13.013) (-41.7427, -12.9238) (-41.6297, -12.6372) (-41.6503, -12.4031) knots 0 0 0 1 2 2 2
  spline S193 degree 2 poles (-41.6503, -12.4031) (-41.671, -12.169) (-41.965, -11.6947) (-42.1878, -11.4743) knots 0 0 0 1 2 2 2
  line L121 (-42.1878, -11.4743) -> (-44.9809, -11.7207)
  line L122 (-44.9809, -11.7207) -> (-45.0364, -11.091)
  line L123 (-45.0364, -11.091) -> (-41.2989, -10.7614)
  line L124 (-41.2989, -10.7614) -> (-41.2433, -11.391)
  line L125 (-41.2433, -11.391) -> (-41.6591, -11.4277)
  spline S194 degree 2 poles (-41.6591, -11.4277) (-41.3799, -11.6878) (-41.0654, -12.2092) (-41.0384, -12.5159) knots 0 0 0 1 2 2 2
  spline S195 degree 2 poles (-41.0384, -12.5159) (-40.9899, -13.0649) (-41.6616, -13.7505) (-42.3518, -13.8114) knots 0 0 0 1 2 2 2
  line L126 (-42.3518, -13.8114) -> (-44.7776, -14.0253)
  line L127 (-44.3556, -17.7738) -> (-44.4282, -17.1459)
  line L128 (-44.4282, -17.1459) -> (-44.0499, -17.1022)
  spline S196 degree 2 poles (-44.0499, -17.1022) (-44.1874, -16.9712) (-44.3731, -16.7765) (-44.4583, -16.6395) knots 0 0 0 1 2 2 2
  spline S197 degree 2 poles (-44.4583, -16.6395) (-44.538, -16.5141) (-44.6395, -16.2363) (-44.6614, -16.0471) knots 0 0 0 1 2 2 2
  spline S198 degree 2 poles (-44.6614, -16.0471) (-44.6967, -15.7412) (-44.5027, -15.1967) (-44.2781, -14.9872) knots 0 0 0 1 2 2 2
  spline S199 degree 2 poles (-44.2781, -14.9872) (-44.0536, -14.7776) (-43.3523, -14.4926) (-42.8814, -14.4381) knots 0 0 0 1 2 2 2
  spline S200 degree 2 poles (-42.8814, -14.4381) (-42.3903, -14.3814) (-41.6446, -14.5521) (-41.3493, -14.7423) knots 0 0 0 1 2 2 2
  spline S201 degree 2 poles (-41.3493, -14.7423) (-41.084, -14.9196) (-40.7398, -15.4631) (-40.703, -15.7811) knots 0 0 0 1 2 2 2
  spline S202 degree 2 poles (-40.703, -15.7811) (-40.6709, -16.0588) (-40.7477, -16.4878) (-40.85, -16.7321) knots 0 0 0 1 2 2 2
  line L129 (-40.85, -16.7321) -> (-39.24, -16.546)
  line L130 (-39.24, -16.546) -> (-39.1674, -17.1739)
  line L131 (-39.1674, -17.1739) -> (-44.3556, -17.7738)
  line L132 (-43.5226, -17.0412) -> (-41.3692, -16.7922)
  spline S203 degree 2 poles (-41.3692, -16.7922) (-41.2835, -16.5457) (-41.2418, -16.1656) (-41.2665, -15.9523) knots 0 0 0 1 2 2 2
  spline S204 degree 2 poles (-41.2665, -15.9523) (-41.3223, -15.4693) (-42.1101, -15.0057) (-42.7944, -15.0848) knots 0 0 0 1 2 2 2
  spline S205 degree 2 poles (-42.7944, -15.0848) (-43.4545, -15.1611) (-44.1024, -15.6602) (-44.0489, -16.1231) knots 0 0 0 1 2 2 2
  spline S206 degree 2 poles (-44.0489, -16.1231) (-44.0205, -16.3686) (-43.7374, -16.8417) (-43.5226, -17.0412) knots 0 0 0 1 2 2 2
  spline S207 degree 2 poles (-39.2724, -21.3403) (-39.301, -21.1602) (-39.4455, -20.818) (-39.5408, -20.6567) knots 0 0 0 1 2 2 2
  spline S208 degree 2 poles (-39.5408, -20.6567) (-39.6342, -20.5074) (-39.8157, -20.2941) (-39.8944, -20.2122) knots 0 0 0 1 2 2 2
  line L133 (-39.8944, -20.2122) -> (-39.9007, -20.1722)
  line L134 (-39.9007, -20.1722) -> (-39.2004, -20.0612)
  spline S209 degree 2 poles (-39.2004, -20.0612) (-39.0501, -20.2589) (-38.7446, -20.9694) (-38.6919, -21.3015) knots 0 0 0 1 2 2 2
  spline S210 degree 2 poles (-38.6919, -21.3015) (-38.6386, -21.6377) (-38.6953, -22.1595) (-38.8071, -22.3864) knots 0 0 0 1 2 2 2
  spline S211 degree 2 poles (-38.8071, -22.3864) (-38.9289, -22.6273) (-39.3455, -22.9231) (-39.6497, -22.9713) knots 0 0 0 1 2 2 2
  spline S212 degree 2 poles (-39.6497, -22.9713) (-40.0579, -23.0361) (-40.7592, -22.5975) (-40.8989, -22.2341) knots 0 0 0 1 2 2 2
  line L135 (-40.8989, -22.2341) -> (-40.9469, -22.2417)
  spline S213 degree 2 poles (-40.9469, -22.2417) (-40.9542, -22.4028) (-41.0417, -22.7818) (-41.1617, -22.9567) knots 0 0 0 1 2 2 2
  spline S214 degree 2 poles (-41.1617, -22.9567) (-41.2777, -23.131) (-41.6954, -23.3942) (-42.0196, -23.4456) knots 0 0 0 1 2 2 2
  spline S215 degree 2 poles (-42.0196, -23.4456) (-42.3517, -23.4983) (-42.9521, -23.3596) (-43.2012, -23.1858) knots 0 0 0 1 2 2 2
  spline S216 degree 2 poles (-43.2012, -23.1858) (-43.4596, -23.0052) (-43.7888, -22.4298) (-43.8504, -22.0416) knots 0 0 0 1 2 2 2
  spline S217 degree 2 poles (-43.8504, -22.0416) (-43.9094, -21.6694) (-43.8448, -20.9125) (-43.7601, -20.6447) knots 0 0 0 1 2 2 2
  line L136 (-43.7601, -20.6447) -> (-43.0598, -20.5337)
  line L137 (-43.0598, -20.5337) -> (-43.0521, -20.5817)
  spline S218 degree 2 poles (-43.0521, -20.5817) (-43.1712, -20.8139) (-43.3397, -21.5627) (-43.2844, -21.9108) knots 0 0 0 1 2 2 2
  spline S219 degree 2 poles (-43.2844, -21.9108) (-43.2521, -22.1149) (-43.0593, -22.5028) (-42.8896, -22.6154) knots 0 0 0 1 2 2 2
  spline S220 degree 2 poles (-42.8896, -22.6154) (-42.7206, -22.724) (-42.3463, -22.8082) (-42.0781, -22.7657) knots 0 0 0 1 2 2 2
  spline S221 degree 2 poles (-42.0781, -22.7657) (-41.81, -22.7232) (-41.4866, -22.5119) (-41.4088, -22.3559) knots 0 0 0 1 2 2 2
  spline S222 degree 2 poles (-41.4088, -22.3559) (-41.3309, -22.2) (-41.3152, -21.8078) (-41.3507, -21.5837) knots 0 0 0 1 2 2 2
  line L138 (-41.3507, -21.5837) -> (-41.3951, -21.3035)
  line L139 (-41.3951, -21.3035) -> (-40.8469, -21.2166)
  line L140 (-40.8469, -21.2166) -> (-40.812, -21.4367)
  spline S223 degree 2 poles (-40.812, -21.4367) (-40.7415, -21.8809) (-40.2285, -22.3739) (-39.8243, -22.3098) knots 0 0 0 1 2 2 2
  spline S224 degree 2 poles (-39.8243, -22.3098) (-39.6362, -22.28) (-39.3909, -22.0934) (-39.3293, -21.9647) knots 0 0 0 1 2 2 2
  spline S225 degree 2 poles (-39.3293, -21.9647) (-39.2649, -21.8273) (-39.2451, -21.5123) (-39.2724, -21.3403) knots 0 0 0 1 2 2 2
  spline S226 degree 2 poles (-41.2407, -27.1097) (-41.5952, -27.1756) (-42.243, -27.0612) (-42.5046, -26.8956) knots 0 0 0 1 2 2 2
  spline S227 degree 2 poles (-42.5046, -26.8956) (-42.7662, -26.73) (-43.14, -26.1607) (-43.2111, -25.7783) knots 0 0 0 1 2 2 2
  spline S228 degree 2 poles (-43.2111, -25.7783) (-43.2764, -25.4277) (-43.2485, -24.7137) (-43.1717, -24.4397) knots 0 0 0 1 2 2 2
  line L141 (-43.1717, -24.4397) -> (-42.4746, -24.31)
  line L142 (-42.4746, -24.31) -> (-42.4657, -24.3578)
  spline S229 degree 2 poles (-42.4657, -24.3578) (-42.5074, -24.4439) (-42.5982, -24.7534) (-42.63, -24.9365) knots 0 0 0 1 2 2 2
  spline S230 degree 2 poles (-42.63, -24.9365) (-42.6614, -25.1443) (-42.6771, -25.4811) (-42.6393, -25.6842) knots 0 0 0 1 2 2 2
  spline S231 degree 2 poles (-42.6393, -25.6842) (-42.6022, -25.8834) (-42.3892, -26.2312) (-42.2086, -26.3377) knots 0 0 0 1 2 2 2
  spline S232 degree 2 poles (-42.2086, -26.3377) (-42.0382, -26.4338) (-41.6241, -26.4886) (-41.3612, -26.4397) knots 0 0 0 1 2 2 2
  spline S233 degree 2 poles (-41.3612, -26.4397) (-41.0983, -26.3908) (-40.7904, -26.1851) (-40.704, -26.0289) knots 0 0 0 1 2 2 2
  spline S234 degree 2 poles (-40.704, -26.0289) (-40.6065, -25.8665) (-40.58, -25.433) (-40.6267, -25.182) knots 0 0 0 1 2 2 2
  spline S235 degree 2 poles (-40.6267, -25.182) (-40.6771, -24.9111) (-40.8608, -24.3889) (-40.927, -24.2323) knots 0 0 0 1 2 2 2
  line L143 (-40.927, -24.2323) -> (-38.3935, -23.7609)
  line L144 (-38.3935, -23.7609) -> (-37.8918, -26.4577)
  line L145 (-37.8918, -26.4577) -> (-38.4694, -26.5652)
  line L146 (-38.4694, -26.5652) -> (-38.8533, -24.5017)
  line L147 (-38.8533, -24.5017) -> (-40.1639, -24.7456)
  spline S236 degree 2 poles (-40.1639, -24.7456) (-40.1257, -24.8621) (-40.0708, -25.0909) (-40.053, -25.1866) knots 0 0 0 1 2 2 2
  spline S237 degree 2 poles (-40.053, -25.1866) (-39.9826, -25.565) (-40.009, -26.1098) (-40.1477, -26.3829) knots 0 0 0 1 2 2 2
  spline S238 degree 2 poles (-40.1477, -26.3829) (-40.2858, -26.66) (-40.7945, -27.0267) (-41.2407, -27.1097) knots 0 0 0 1 2 2 2
  line L148 (-41.7354, -32.3551) -> (-39.6149, -31.8857)
  spline S239 degree 2 poles (-39.6149, -31.8857) (-39.3617, -31.8297) (-38.9393, -31.6947) (-38.8346, -31.6051) knots 0 0 0 1 2 2 2
  spline S240 degree 2 poles (-38.8346, -31.6051) (-38.718, -31.5129) (-38.6449, -31.2436) (-38.6913, -31.0339) knots 0 0 0 1 2 2 2
  spline S241 degree 2 poles (-38.6913, -31.0339) (-38.7333, -30.844) (-39.063, -30.4605) (-39.3354, -30.2801) knots 0 0 0 1 2 2 2
  spline S242 degree 2 poles (-39.3354, -30.2801) (-39.3899, -30.2963) (-39.5424, -30.3383) (-39.6453, -30.3611) knots 0 0 0 1 2 2 2
  line L149 (-39.6453, -30.3611) -> (-42.0585, -30.8953)
  line L150 (-42.0585, -30.8953) -> (-42.1951, -30.2781)
  line L151 (-42.1951, -30.2781) -> (-40.0746, -29.8088)
  spline S243 degree 2 poles (-40.0746, -29.8088) (-39.8214, -29.7527) (-39.399, -29.6177) (-39.2943, -29.5281) knots 0 0 0 1 2 2 2
  spline S244 degree 2 poles (-39.2943, -29.5281) (-39.1778, -29.4359) (-39.1046, -29.1666) (-39.151, -28.9569) knots 0 0 0 1 2 2 2
  spline S245 degree 2 poles (-39.151, -28.9569) (-39.1948, -28.7591) (-39.5412, -28.3752) (-39.7806, -28.2123) knots 0 0 0 1 2 2 2
  line L152 (-39.7806, -28.2123) -> (-42.5182, -28.8183)
  line L153 (-42.5182, -28.8183) -> (-42.6548, -28.2012)
  line L154 (-42.6548, -28.2012) -> (-38.9915, -27.3903)
  line L155 (-38.9915, -27.3903) -> (-38.8549, -28.0074)
  line L156 (-38.8549, -28.0074) -> (-39.2584, -28.0968)
  spline S246 degree 2 poles (-39.2584, -28.0968) (-38.9637, -28.2847) (-38.5935, -28.7007) (-38.5305, -28.9856) knots 0 0 0 1 2 2 2
  spline S247 degree 2 poles (-38.5305, -28.9856) (-38.4587, -29.31) (-38.6442, -29.8781) (-38.9515, -30.0831) knots 0 0 0 1 2 2 2
  spline S248 degree 2 poles (-38.9515, -30.0831) (-38.5768, -30.2948) (-38.139, -30.754) (-38.0707, -31.0625) knots 0 0 0 1 2 2 2
  spline S249 degree 2 poles (-38.0707, -31.0625) (-38.0182, -31.2999) (-38.0788, -31.72) (-38.2134, -31.8992) knots 0 0 0 1 2 2 2
  spline S250 degree 2 poles (-38.2134, -31.8992) (-38.3472, -32.0823) (-38.8097, -32.3549) (-39.1856, -32.4381) knots 0 0 0 1 2 2 2
  line L157 (-39.1856, -32.4381) -> (-41.5988, -32.9722)
  line L158 (-41.5988, -32.9722) -> (-41.7354, -32.3551)
  line L159 (-40.2995, -37.9468) -> (-38.2001, -37.3908)
  spline S251 degree 2 poles (-38.2001, -37.3908) (-37.9494, -37.3244) (-37.5329, -37.1722) (-37.432, -37.0784) knots 0 0 0 1 2 2 2
  spline S252 degree 2 poles (-37.432, -37.0784) (-37.3193, -36.9815) (-37.2572, -36.7094) (-37.3122, -36.5018) knots 0 0 0 1 2 2 2
  spline S253 degree 2 poles (-37.3122, -36.5018) (-37.362, -36.3138) (-37.7072, -35.9441) (-37.9867, -35.775) knots 0 0 0 1 2 2 2
  spline S254 degree 2 poles (-37.9867, -35.775) (-38.0405, -35.7935) (-38.1912, -35.8418) (-38.293, -35.8687) knots 0 0 0 1 2 2 2
  line L160 (-38.293, -35.8687) -> (-40.6823, -36.5015)
  line L161 (-40.6823, -36.5015) -> (-40.8441, -35.8905)
  line L162 (-40.8441, -35.8905) -> (-38.7447, -35.3345)
  spline S255 degree 2 poles (-38.7447, -35.3345) (-38.494, -35.2681) (-38.0775, -35.1159) (-37.9766, -35.0221) knots 0 0 0 1 2 2 2
  spline S256 degree 2 poles (-37.9766, -35.0221) (-37.8639, -34.9252) (-37.8019, -34.653) (-37.8568, -34.4454) knots 0 0 0 1 2 2 2
  spline S257 degree 2 poles (-37.8568, -34.4454) (-37.9087, -34.2496) (-38.2706, -33.8802) (-38.5165, -33.7273) knots 0 0 0 1 2 2 2
  line L163 (-38.5165, -33.7273) -> (-41.2269, -34.4452)
  line L164 (-41.2269, -34.4452) -> (-41.3887, -33.8342)
  line L165 (-41.3887, -33.8342) -> (-37.7618, -32.8736)
  line L166 (-37.7618, -32.8736) -> (-37.5999, -33.4846)
  line L167 (-37.5999, -33.4846) -> (-37.9995, -33.5904)
  spline S258 degree 2 poles (-37.9995, -33.5904) (-37.6972, -33.7661) (-37.3103, -34.1666) (-37.2356, -34.4486) knots 0 0 0 1 2 2 2
  spline S259 degree 2 poles (-37.2356, -34.4486) (-37.1506, -34.7698) (-37.3126, -35.345) (-37.6113, -35.5624) knots 0 0 0 1 2 2 2
  spline S260 degree 2 poles (-37.6113, -35.5624) (-37.2282, -35.7586) (-36.772, -36.1994) (-36.691, -36.5049) knots 0 0 0 1 2 2 2
  spline S261 degree 2 poles (-36.691, -36.5049) (-36.6288, -36.7399) (-36.6721, -37.1622) (-36.7992, -37.3467) knots 0 0 0 1 2 2 2
  spline S262 degree 2 poles (-36.7992, -37.3467) (-36.9253, -37.5352) (-37.3763, -37.8265) (-37.7484, -37.9251) knots 0 0 0 1 2 2 2
  line L168 (-37.7484, -37.9251) -> (-40.1377, -38.5579)
  line L169 (-40.1377, -38.5579) -> (-40.2995, -37.9468)
  spline S263 degree 2 poles (-36.4266, -43.8606) (-37.3223, -44.1458) (-38.6519, -43.6294) (-38.8596, -42.9769) knots 0 0 0 1 2 2 2
  spline S264 degree 2 poles (-38.8596, -42.9769) (-38.9444, -42.7105) (-38.9512, -42.2619) (-38.8914, -42.009) knots 0 0 0 1 2 2 2
  line L170 (-38.8914, -42.009) -> (-40.3894, -42.4859)
  line L171 (-40.3894, -42.4859) -> (-40.5812, -41.8836)
  line L172 (-40.5812, -41.8836) -> (-35.6894, -40.3262)
  line L173 (-35.6894, -40.3262) -> (-35.4976, -40.9285)
  line L174 (-35.4976, -40.9285) -> (-35.8721, -41.0477)
  spline S265 degree 2 poles (-35.8721, -41.0477) (-35.5962, -41.2065) (-35.1514, -41.6687) (-35.0494, -41.9891) knots 0 0 0 1 2 2 2
  spline S266 degree 2 poles (-35.0494, -41.9891) (-34.8539, -42.603) (-35.6081, -43.6) (-36.4266, -43.8606) knots 0 0 0 1 2 2 2
  spline S267 degree 2 poles (-36.694, -43.2611) (-36.0801, -43.0657) (-35.5286, -42.4606) (-35.6675, -42.0244) knots 0 0 0 1 2 2 2
  spline S268 degree 2 poles (-35.6675, -42.0244) (-35.7486, -41.7695) (-36.1288, -41.3633) (-36.3741, -41.2075) knots 0 0 0 1 2 2 2
  line L175 (-36.3741, -41.2075) -> (-38.4049, -41.8541)
  spline S269 degree 2 poles (-38.4049, -41.8541) (-38.4419, -42.1252) (-38.4199, -42.4882) (-38.351, -42.7044) knots 0 0 0 1 2 2 2
  spline S270 degree 2 poles (-38.351, -42.7044) (-38.2023, -43.1716) (-37.3503, -43.4701) (-36.694, -43.2611) knots 0 0 0 1 2 2 2
  spline S271 degree 2 poles (-37.6444, -46.6482) (-37.9398, -45.7986) (-37.3115, -44.5334) (-36.4313, -44.2274) knots 0 0 0 1 2 2 2
  spline S272 degree 2 poles (-36.4313, -44.2274) (-35.5664, -43.9266) (-34.2253, -44.4771) (-33.9712, -45.208) knots 0 0 0 1 2 2 2
  spline S273 degree 2 poles (-33.9712, -45.208) (-33.8567, -45.5372) (-33.8711, -46.1127) (-34.0088, -46.3708) knots 0 0 0 1 2 2 2
  spline S274 degree 2 poles (-34.0088, -46.3708) (-34.1451, -46.6327) (-34.6601, -47.0391) (-35.0849, -47.1868) knots 0 0 0 1 2 2 2
  line L176 (-35.0849, -47.1868) -> (-35.4102, -47.2999)
  line L177 (-35.4102, -47.2999) -> (-36.2632, -44.8467)
  spline S275 degree 2 poles (-36.2632, -44.8467) (-36.8793, -45.0609) (-37.3182, -45.9085) (-37.1266, -46.4596) knots 0 0 0 1 2 2 2
  spline S276 degree 2 poles (-37.1266, -46.4596) (-37.0587, -46.6548) (-36.839, -47.003) (-36.7168, -47.1322) knots 0 0 0 1 2 2 2
  spline S277 degree 2 poles (-36.7168, -47.1322) (-36.5844, -47.2663) (-36.3733, -47.4417) (-36.2868, -47.4931) knots 0 0 0 1 2 2 2
  line L178 (-36.2868, -47.4931) -> (-36.2748, -47.5276)
  line L179 (-36.2748, -47.5276) -> (-36.9254, -47.7538)
  spline S278 degree 2 poles (-36.9254, -47.7538) (-37.0034, -47.6651) (-37.235, -47.3939) (-37.312, -47.2834) knots 0 0 0 1 2 2 2
  spline S279 degree 2 poles (-37.312, -47.2834) (-37.4217, -47.1284) (-37.5699, -46.8625) (-37.6444, -46.6482) knots 0 0 0 1 2 2 2
  spline S280 degree 2 poles (-35.157, -46.5598) (-34.9186, -46.4683) (-34.6011, -46.2464) (-34.5157, -46.1095) knots 0 0 0 1 2 2 2